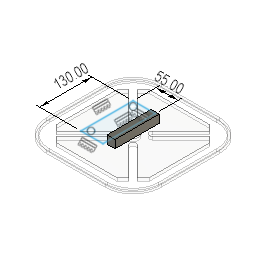
Adaptador+Taladro+de+Columna (Autodesk Fusion 360 design; units mm, degrees)
Autodesk Fusion 360 part; units mm, degrees
sketch "Sketch1" plane through (0, 0, 0) normal (0, 0, 1) x (1, 0, 0) in component "Base Taladro"
  line L0 (40, 0) -> (190, 0)
  line L1 (230, 40) -> (230, 190)
  line L2 (190, 230) -> (40, 230)
  line L3 (0, 190) -> (0, 40)
  line L4 (230, 190) -> (190, 230)
  line L5 (40, 230) -> (0, 190)
  line L6 (190, 0) -> (230, 40)
  line L7 (40, 0) -> (0, 40)
  line L8 (20, 210) -> (210, 20) construction
  line L9 (20, 20) -> (210, 210) construction
  circle A0 centre (115, 115) radius 13
  circle A1 centre (115, 115) radius 26.5 construction
  line L10 (96.2617, 133.7383) -> (101.9185, 139.3952) construction
  line L11 (101.9185, 139.3952) -> (120.6569, 120.6569) construction
  line L12 (120.6569, 120.6569) -> (115, 115) construction
  line L13 (115, 115) -> (96.2617, 133.7383) construction
  line L14 (96.2617, 133.7383) -> (90.6048, 128.0815) construction
  line L15 (25.6569, 215.6569) -> (14.3431, 204.3431)
  circle A2 centre (90.6048, 139.3952) radius 8
  line L16 (14.3431, 204.3431) -> (84.948, 133.7383)
  line L17 (25.6569, 215.6569) -> (96.2617, 145.052)
  line L18 (115, 115) -> (115, 264) construction
  line L19 (204.3431, 215.6569) -> (133.7383, 145.052)
  circle A3 centre (139.3952, 139.3952) radius 8
  line L20 (215.6569, 204.3431) -> (145.052, 133.7383)
  line L21 (115, 115) -> (230, 115) construction
  line L22 (14.3431, 25.6569) -> (84.948, 96.2617)
  circle A4 centre (90.6048, 90.6048) radius 8
  line L23 (25.6569, 14.3431) -> (96.2617, 84.948)
  line L24 (204.3431, 14.3431) -> (133.7383, 84.948)
  circle A5 centre (139.3952, 90.6048) radius 8
  line L25 (215.6569, 25.6569) -> (145.052, 96.2617)
  line L26 (187.5, 257.5) -> (42.5, 257.5)
  line L27 (-27.5, 187.5) -> (-27.5, 42.5)
  line L28 (42.5, -27.5) -> (187.5, -27.5)
  line L29 (257.5, 42.5) -> (257.5, 187.5)
  line L30 (257.5, 257.5) -> (-27.5, -27.5) construction
  line L31 (-27.5, 257.5) -> (257.5, -27.5) construction
  arc A6 (42.5, 257.5) -> (-27.5, 187.5) centre (42.5, 187.5) ccw
  arc A7 (257.5, 187.5) -> (187.5, 257.5) centre (187.5, 187.5) ccw
  arc A8 (187.5, -27.5) -> (257.5, 42.5) centre (187.5, 42.5) ccw
  arc A9 (-27.5, 42.5) -> (42.5, -27.5) centre (42.5, 42.5) ccw
  line L32 (-21.5, 187.5) -> (-21.5, 42.5)
  arc A10 (-21.5, 42.5) -> (42.5, -21.5) centre (42.5, 42.5) ccw
  line L33 (42.5, -21.5) -> (187.5, -21.5)
  arc A11 (187.5, -21.5) -> (251.5, 42.5) centre (187.5, 42.5) ccw
  line L34 (251.5, 42.5) -> (251.5, 187.5)
  arc A12 (251.5, 187.5) -> (187.5, 251.5) centre (187.5, 187.5) ccw
  line L35 (187.5, 251.5) -> (42.5, 251.5)
  arc A13 (42.5, 251.5) -> (-21.5, 187.5) centre (42.5, 187.5) ccw
  point P0 (230, 0)
  point P1 (230, 230)
  point P2 (0, 230)
  point P3 (115, 115)
  dimension "d1" = 230
  dimension "d2" = 230
  dimension "d3" = 40
  dimension "d4" = 40
  dimension "d5" = 40
  dimension "d6" = 40
  dimension "d8" = 40
  dimension "d9" = 40
  dimension "d10" = 40
  dimension "d11" = 40
  dimension "d13" = 26
  dimension "d14" = 53
  dimension "d15" = 8
  dimension "d16" = 8
  dimension "d17" = 16
  dimension "d18" = 8
  dimension "d25" = 285
  dimension "d26" = 285
  dimension "d27" = 70
  dimension "d28" = 70
  dimension "d29" = 70
  dimension "d30" = 70
  dimension "d31" = -6
  constraint horizontal L0
  constraint vertical L1
  constraint horizontal L2
  constraint vertical L3
  constraint coincident P1 L1
  constraint coincident P1 L2
  constraint coincident P2 L2
  constraint coincident P2 L3
  constraint coincident P0 L0
  constraint coincident P0 L1
  constraint coincident origin L0
  constraint coincident origin L3
  constraint midpoint L5 L8.start
  constraint midpoint L6 L8.end
  constraint midpoint L7 L9.start
  constraint midpoint L4 L9.end
  constraint midpoint L8 P3
  constraint concentric A0 A1
  constraint perpendicular L10 L11
  constraint parallel L10 L12
  constraint parallel L11 L13
  constraint perpendicular L8 L10
  constraint coincident A1 L10.start
  constraint coincident L8 L10.start
  constraint perpendicular L8 L14
  constraint coincident A2 L16.end
  constraint tangent A2 L16
  constraint perpendicular L5 L16
  constraint coincident A2 L17.end
  constraint tangent A2 L17
  constraint perpendicular L5 L17
  constraint coincident P3 A0.centre
  constraint vertical L18
  constraint symmetric L15.start L18 L19.start
  constraint symmetric L15.end L18 L20.start
  constraint symmetric A2 L18 A3
  constraint symmetric L16.end L18 L20.end
  constraint symmetric L17.end L18 L19.end
  constraint midpoint L1 L21.end
  constraint symmetric L15.start L21 L23.start
  constraint symmetric L15.end L21 L22.start
  constraint symmetric A2 L21 A4
  constraint symmetric L16.end L21 L22.end
  constraint symmetric L17.end L21 L23.end
  constraint symmetric L19.start L21 L24.start
  constraint symmetric L19.end L21 L24.end
  constraint symmetric A3 L21 A5
  constraint symmetric L20.start L21 L25.start
  constraint symmetric L20.end L21 L25.end
  constraint horizontal L26
  constraint perpendicular L26 L27
  constraint parallel L26 L28
  constraint parallel L27 L29
  constraint coincident L30 P3
  constraint coincident L31 P3
  constraint coincident L31.start L26
  constraint coincident L31.start L27
  constraint tangent L26 A6
  constraint tangent L27 A6
  constraint coincident L30.start L26
  constraint coincident L30.start L29
  constraint tangent L26 A7
  constraint tangent L29 A7
  constraint coincident L31.end L28
  constraint coincident L31.end L29
  constraint tangent L28 A8
  constraint tangent L29 A8
  constraint coincident L30.end L28
  constraint coincident L30.end L27
  constraint tangent L28 A9
  constraint tangent L27 A9
  measures "d1" distance of origin P0
  measures "d2" distance of origin P2
  measures "d3" distance of P1 L1.end
  measures "d4" distance of P1 L2.start
  measures "d5" distance of P2 L2.end
  measures "d6" distance of P2 L3.start
  measures "d8" distance of P0 L0.end
  measures "d9" distance of P0 L1.start
  measures "d10" distance of origin L0.start
  measures "d11" distance of origin L3.end
  measures "d13" diameter of A0
  measures "d14" diameter of A1
  measures "d15" distance of L10.start L10.end
  measures "d16" distance of L10.start L14.end
  measures "d17" distance of L15.start L15.end
  measures "d18" radius of A2
  measures "d25" distance of L30.end L31.end
  measures "d26" distance of L31.start L30.end
  measures "d27" radius of A6
  measures "d28" radius of A7
  measures "d29" radius of A8
  measures "d30" radius of A9
extrude "Extrude1" add sketch "Sketch1" along normal blind 8 contours L0 L1 L2 L3 L4 L5 L6 L7 A2 L16 L17 L19 A3 L20 L22 A4 L23 L24 A5 L25 makes body 1
fillet "Fillet1" radius 1.5 1 edges at (102.8797, 119.701, 8) on bodies 1
fillet "Fillet2" radius 0.1 24 edges at (197.1716, 222.8284, 8) (115, 230, 8) (32.8284, 222.8284, 8) (60.9593, 180.3544, 8) (96.2617, 133.7383, 8) (49.6456, 169.0407, 8) (7.1716, 197.1716, 8) (0, 115, 8) (7.1716, 32.8284, 8) (32.8284, 7.1716, 8) (49.6456, 60.9593, 8) (96.2617, 96.2617, 8) (60.9593, 49.6456, 8) (115, 0, 8) (197.1716, 7.1716, 8) (169.0407, 49.6456, 8) (133.7383, 96.2617, 8) (180.3544, 60.9593, 8) (222.8284, 32.8284, 8) (230, 115, 8) (222.8284, 197.1716, 8) (180.3544, 169.0407, 8) (133.7383, 133.7383, 8) (169.0407, 180.3544, 8) on bodies 1
copy_body "CutPasteBodies1" bodies 1 removing the originals makes body 2 in component "Base Taladro"
extrude "Extrude1'" add sketch "Sketch1" along normal blind 8 separate body contours L26 L27 L28 L29 A6 A7 A8 A9 makes body 3 in component "Base Taladro"
sketch "base madera" plane through (0, 0, 8) normal (0, 0, 1) x (-1, 0, 0) in component "Base Madera"
  line L0 (-30, -200) -> (-200, -200)
  line L1 (-200, -200) -> (-200, -30)
  line L2 (-200, -30) -> (-30, -30)
  line L3 (-30, -30) -> (-30, -200)
  circle A0 centre (-62.5269, -167.4731) radius 6.5
  circle A1 centre (-167.4731, -167.4731) radius 6.5
  circle A2 centre (-62.5269, -62.5269) radius 6.5
  circle A3 centre (-167.4731, -62.5269) radius 6.5
  circle A4 centre (-115, -115) radius 13
  point P0 (-115, -115)
  dimension "d39" = 26
  dimension "d40" = 46
  dimension "d41" = 170
  dimension "d42" = 170
  dimension "d45" = 13
  constraint horizontal L0
  constraint perpendicular L0 L1
  constraint parallel L0 L2
  constraint parallel L1 L3
  measures "d39" diameter of A4
  measures "d40" distance of L0.start A0.centre
  measures "d41" distance of L0.start L0.end
  measures "d42" distance of L0.end L1.end
  measures "d45" diameter of A1
sketch "perfil" plane through (0, 0, 0) normal (0, 0, 1) x (1, 0, 0) in component "Base Madera"
  line L0 (125, 170, 8) -> (105, 170, 8)
  line L1 (105, 170, 8) -> (105, 60, 8)
  line L2 (105, 60, 8) -> (125, 60, 8)
  line L3 (125, 60, 8) -> (125, 170, 8)
  line L4 (125, 170, 8) -> (105, 60, 8) construction
  line L5 (105, 170, 8) -> (125, 60, 8) construction
  point P0 (115, 115)
  dimension "d46" = 20
  dimension "d47" = 110
extrude "Extrude1''" add sketch "perfil" along normal blind 20 separate body contours L0 L1 L2 L3 in plane through (0, 0, 8) normal (0, 0, 1) makes body 4 in component "Base Madera"
sketch "pernos madera" plane through (0, 0, 8) normal (0, 0, 1) x (-1, 0, 0) in component "Base Madera"
  line L0 (-105, -180, 6) -> (-50, -180, 6)
  line L1 (-50, -180, 6) -> (-50, -50, 6)
  line L2 (-50, -50, 6) -> (-105, -50, 6)
  line L3 (-105, -50, 6) -> (-105, -180, 6)
  circle A0 through (-56.0269, -167.4731, 6) (-65.7769, -161.8439, 6) (-65.7769, -173.1023, 6)
  circle A1 through (-56.0269, -62.5269, 6) (-65.7769, -56.8977, 6) (-65.7769, -68.1561, 6)
  dimension "d62" = 55
  dimension "d63" = 130
extrude "Extrude2" [rolled back] along distance 6 taper angle 0 in component "Base Madera"
extrude "Extrude3" [rolled back] along distance 6 taper angle 0 in component "Base Madera"
scale "Scale1" [rolled back] in component "Base Madera"
move_body "Move1" [rolled back] translate x 0 translate y 0 translate z 6 in component "Base Madera"
component "Base Madera" placed x (1, 0, 0) y (0, 1, 0) z (0, 0, 1) at (0, 0, 0)
component "Base Taladro" placed x (1, 0, 0) y (0, 1, 0) z (0, 0, 1) at (0, 0, 0)
equation "d4 = d3"
equation "d6 = d5"
equation "d9 = d8"
equation "d11 = d10"
equation "d14 = 26 mm + 27 mm"
named bodies: "perfil", "base madera", "perno"
